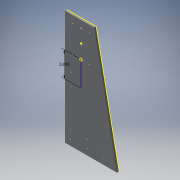
# Autodesk Inventor part: Side Walls
Saved by Autodesk Inventor 2016 (Build 200138000, 138)
## iProperties
Created: 2016-04-23
Part Number: Side Walls
Material: Generic
Document SubType Name: Modeling
Designer: Scott
Density: 1 g/cm^3
Appearance: Default
Author: Scott
Autodesk Inventor part; units mm, degrees
ref_plane "YZ Plane" through (0, 0, 0) normal (1, 0, 0) x (0, 1, 0)
ref_plane "XZ Plane" through (0, 0, 0) normal (0, 1, 0) x (-1, 0, 0)
ref_plane "XY Plane" through (0, 0, 0) normal (0, 0, 1) x (1, 0, 0)
ref_plane "Work Plane1" through (-0.1788, 0, 0) normal (0, 0, 1) x (1, 0, 0)
sketch "Sketch1" plane through (-0.1788, 0, 0) normal (0, 0, 1) x (1, 0, 0)
  line L0 (-15.3244, 3.4987) -> (-19.1223, 3.4987) projected
  line L1 (-19.1223, 3.4987) -> (-28.8529, 35.0248) projected
  arc A0 (-28.8529, 35.0248) -> (-20.5467, 47.7802) centre (-25.0147, 41.6076) ccw projected
  line L2 (-20.5467, 47.7802) -> (-6.566, 47.7802) projected
  arc A1 (-6.566, 47.7802) -> (-2.0556, 33.1897) centre (0.3832, 41.936) ccw projected
  line L3 (-2.0556, 33.1897) -> (-2.0556, 15.9522) projected
  arc A2 (-2.0556, 15.9522) -> (-15.3244, 3.4987) centre (0.3832, 0.0582) ccw projected
  arc A3 (20.8934, 47.7802) -> (21.5632, 35.5913) centre (25.7832, 41.936) ccw projected
  line L4 (21.5632, 35.5913) -> (21.5632, 4.0758) projected
  line L5 (21.5632, 4.0758) -> (15.9532, 4.0758) projected
  arc A4 (15.9532, 4.0758) -> (1.9969, 16.0571) centre (0.3832, 0.0582) ccw projected
  line L6 (1.9969, 16.0571) -> (1.9969, 33.0006) projected
  arc A5 (1.9969, 33.0006) -> (7.3324, 47.7802) centre (0.3832, 41.936) ccw projected
  line L7 (7.3324, 47.7802) -> (20.8934, 47.7802) projected
  arc A6 (21.5632, -35.3114) -> (21.3082, -47.8332) centre (25.7764, -41.6607) ccw projected
  line L8 (21.3082, -47.8332) -> (7.1864, -47.8332) projected
  arc A7 (7.1864, -47.8332) -> (1.9969, -32.8841) centre (0.3832, -41.8196) ccw projected
  line L9 (1.9969, -32.8841) -> (1.9969, -15.9406) projected
  arc A8 (1.9969, -15.9406) -> (16.068, -3.4851) centre (0.3832, 0.0582) ccw projected
  line L10 (16.068, -3.4851) -> (21.5632, -3.4851) projected
  line L11 (21.5632, -3.4851) -> (21.5632, -35.3114) projected
  arc A9 (-20.9828, -47.8332) -> (-29.9021, -35.476) centre (-25.464, -41.6702) ccw projected
  line L12 (-29.9021, -35.476) -> (-19.2115, -3.4851) projected
  line L13 (-19.2115, -3.4851) -> (-15.3016, -3.4851) projected
  arc A10 (-15.3016, -3.4851) -> (-2.0556, -15.8358) centre (0.3832, 0.0582) ccw projected
  line L14 (-2.0556, -15.8358) -> (-2.0556, -33.0732) projected
  arc A11 (-2.0556, -33.0732) -> (-6.4199, -47.8332) centre (0.3832, -41.8196) ccw projected
  line L15 (-6.4199, -47.8332) -> (-20.9828, -47.8332) projected
  circle A12 centre (0.3832, 0.0582) radius 11 projected
  circle A13 centre (0.3832, -41.8196) radius 4 projected
  circle A14 centre (0.3832, 41.936) radius 4 projected
  circle A15 centre (-25.464, -41.6702) radius 2.54 projected
  circle A16 centre (-25.0147, 41.6076) radius 2.54 projected
  circle A17 centre (25.7764, -41.6607) radius 2.54 projected
  circle A18 centre (25.7832, 41.936) radius 2.54 projected
  arc A19 (25.7764, 31.8658) -> (25.2733, 51.9934) centre (25.7832, 41.936) ccw projected
  line L16 (25.2733, 51.9934) -> (-25.0147, 51.9934) projected
  arc A20 (-25.0147, 51.9934) -> (-35.3953, 41.9358) centre (-25.0147, 41.6076) ccw projected
  line L17 (-35.3953, 41.9358) -> (-22.4697, 0.058) projected
  line L18 (-22.4697, 0.058) -> (-35.3142, -38.3784) projected
  arc A21 (-35.3142, -38.3784) -> (-25.0214, -52.0464) centre (-25.464, -41.6702) ccw projected
  line L19 (-25.0214, -52.0464) -> (25.7764, -52.0464) projected
  arc A22 (25.7764, -52.0464) -> (25.7764, -31.275) centre (25.7764, -41.6607) ccw projected
  line L20 (25.7764, -31.275) -> (25.7764, 31.8658) projected
  line L21 (0.1293, 51.9934) -> (0.1293, 62.509)
  line L22 (-35.3953, 41.9358) -> (-48.0953, 41.9358)
  line L23 (-47.8239, 62.509) -> (41.0761, 62.509)
  line L24 (41.0761, 62.509) -> (110.9261, -286.741)
  line L25 (-47.8239, 62.509) -> (-47.8239, -286.741)
  line L26 (-47.8239, -286.741) -> (110.9261, -286.741)
  point P0 (0.1788, 0)
  dimension "d0" = 10.5156
  dimension "d1" = 12.7
  dimension "d4" = 88.9
  dimension "d10" = 349.25
  constraints: 12 end point, 2 vertical, 1 horizontal, 1 midpoint, 1 perpendicular, 1 other
  measures "d0" distance of L21.start L21.end
  measures "d1" distance of L17.start L22.end
  measures "d4" distance of L23.start L23.end
  measures "d10" distance of L23.start L25.end
extrude "Extrusion1" add sketch "Sketch1" along normal blind 6.096 contours L0 L1 A0 L2 A1 L3 A2 | A3 L4 L5 A4 L6 A5 L7 | A6 L8 A7 L9 A8 L10 L11 | A9 L12 L13 A10 L14 A11 L15 | A12 | L20 A22 L19 A21 L18 L17 A20 L16 A19 | A19 L16 L21 L23 L24 L26 L25 L22 L17 L18 A21 L19 A22 L20 | L16 A20 L22 L25 L23 L21
sketch "Sketch2" plane through (-0.1788, 0, 6.096) normal (0, 0, 1) x (1, 0, 0)
  circle A0 centre (0.3832, 0.0582) radius 5 projected
  point P0 (0.1788, 0)
extrude "Extrusion2" cut sketch "Sketch2" against normal blind 25.4
sketch "Sketch3" plane through (-0.1788, 0, 0) normal (0, 0, -1) x (-1, 0, 0)
  circle A0 centre (-0.3832, 0.0582) radius 5 projected
  circle A1 centre (-0.3832, 41.936) radius 4 projected
  circle A2 centre (-0.3832, -41.8196) radius 4 projected
  circle A3 centre (-25.7832, 41.936) radius 2.54 projected
  circle A4 centre (-25.7764, -41.6607) radius 2.54 projected
  circle A5 centre (25.0147, 41.6076) radius 2.54 projected
  circle A6 centre (25.464, -41.6702) radius 2.54 projected
  line L0 (47.8239, 62.509) -> (-41.0761, 62.509) projected
  line L1 (-41.0761, 62.509) -> (-110.9261, -286.741) projected
  line L2 (-110.9261, -286.741) -> (47.8239, -286.741) projected
  line L3 (47.8239, -286.741) -> (47.8239, 62.509) projected
  line L4 (82.12, -280.645) -> (-254.43, -280.645)
  line L5 (-72.5025, -280.645) -> (-68.0575, -280.645)
  line L6 (-21.7025, -280.645) -> (-17.2575, -280.645)
  line L7 (29.0975, -280.645) -> (33.5425, -280.645)
  line L8 (-70.28, -280.645) -> (-70.28, -267.945)
  line L9 (-70.28, -267.945) -> (-19.48, -267.945)
  line L10 (-19.48, -267.945) -> (31.32, -267.945)
  line L11 (31.32, -267.945) -> (31.32, -242.545)
  circle A7 centre (-70.28, -267.945) radius 2.2225
  circle A8 centre (-19.48, -267.945) radius 2.2225
  circle A9 centre (31.32, -267.945) radius 2.2225
  circle A10 centre (31.32, -242.545) radius 2.2225
  circle A11 centre (-19.48, -242.545) radius 2.2225
  circle A12 centre (-70.28, -242.545) radius 2.2225
  point P0 (-0.1788, 0)
  dimension "d11" = 12.7
  dimension "d12" = 25.4
  dimension "d13" = 4.445
  dimension "d14" = 4.445
  dimension "d15" = 4.445
  dimension "d16" = 4.445
  dimension "d17" = 4.445
  dimension "d18" = 4.445
  constraints: 16 end point, 6 centre point, 4 horizontal, 3 coincident, 2 perpendicular, 1 midpoint, 1 point on line, 1 vertical, 8 other
  measures "d11" distance of L8.start L8.end
  measures "d12" distance of L10.end L11.end
  measures "d13" diameter of A7
  measures "d14" diameter of A8
  measures "d15" diameter of A9
  measures "d16" diameter of A10
  measures "d17" diameter of A11
  measures "d18" diameter of A12
extrude "Extrusion3" cut sketch "Sketch3" against normal blind 25.4 contours A10 | A9 L11 L10 | L10 L11 A9 | A8 L10 L9 | L9 L10 A8 | A7 L9 L8 | L8 L9 A7 | A11 | A12
sketch "Sketch4" plane through (-0.1788, 0, 0) normal (0, 0, -1) x (-1, 0, 0)
  circle A0 centre (-19.48, -242.545) radius 2.2225 projected
  circle A1 centre (31.32, -267.945) radius 2.2225 projected
  circle A2 centre (-70.28, -267.945) radius 2.2225 projected
  circle A3 centre (-19.48, -267.945) radius 2.2225 projected
  circle A4 centre (31.32, -242.545) radius 2.2225 projected
  circle A5 centre (-70.28, -242.545) radius 2.2225 projected
  circle A6 centre (-0.3832, 0.0582) radius 5 projected
  circle A7 centre (-0.3832, 41.936) radius 4 projected
  circle A8 centre (-0.3832, -41.8196) radius 4 projected
  circle A9 centre (-25.7832, 41.936) radius 2.54 projected
  circle A10 centre (-25.7764, -41.6607) radius 2.54 projected
  circle A11 centre (25.0147, 41.6076) radius 2.54 projected
  circle A12 centre (25.464, -41.6702) radius 2.54 projected
  line L0 (47.8239, 62.509) -> (-41.0761, 62.509) projected
  line L1 (-41.0761, 62.509) -> (-110.9261, -286.741) projected
  line L2 (-110.9261, -286.741) -> (47.8239, -286.741) projected
  line L3 (47.8239, -286.741) -> (47.8239, 62.509) projected
  point P0 (-0.1788, 0)
sketch "Sketch5" plane through (-0.1788, 0, 6.096) normal (0, 0, 1) x (1, 0, 0)
  circle A0 centre (0.3832, -41.8196) radius 4 projected
  line L0 (0.3832, -41.8196) -> (0.3832, -118.0196)
  point P0 (0.1788, 0)
  dimension "d21" = 76.2
  constraints: 2 end point, 1 vertical
  measures "d21" distance of L0.start L0.end
sketch "Sketch6" plane through (-0.1788, 0, 6.096) normal (0, 0, 1) x (1, 0, 0)
  line L0 (41.0761, 62.509) -> (-47.8239, 62.509) projected
  line L1 (-47.8239, 62.509) -> (-47.8239, -89.891)
  line L2 (-47.8239, 62.509) -> (-47.8239, -286.741) projected
  line L3 (-47.8239, -89.891) -> (-28.7739, -89.891)
  line L4 (-28.7739, -89.891) -> (-28.7739, -127.991)
  circle A0 centre (-28.7739, -89.891) radius 2.2225
  circle A1 centre (-28.7739, -127.991) radius 2.2225
  point P0 (0.1788, 0)
  dimension "d22" = 152.4
  dimension "d23" = 19.05
  dimension "d24" = 38.1
  dimension "d25" = 4.445
  dimension "d26" = 4.445
  constraints: 6 end point, 2 centre point, 2 coincident, 2 perpendicular, 1 point on line
  measures "d22" distance of L0.end L1.end
  measures "d23" distance of L1.end L3.end
  measures "d24" distance of L3.end L4.end
  measures "d25" diameter of A0
  measures "d26" diameter of A1
extrude "Extrusion4" cut sketch "Sketch6" against normal blind 25.4
body "Solid1"
